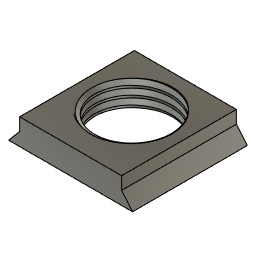
Headset_Hanger_V1.5_Fusion_v2 (Autodesk Fusion 360 archive; units mm, degrees)
design "Headset Hanger Thread"
Autodesk Fusion 360 part; units mm, degrees
sketch "Sketch1" plane through (0, 0, 0) normal (0, 0, 1) x (1, 0, 0)
  line L0 (0, 0) -> (40, 0)
  line L1 (40, 0) -> (40, 10)
  line L2 (40, 10) -> (0, 10)
  line L3 (0, 10) -> (0, 55)
  line L4 (0, 55) -> (40, 55)
  line L5 (40, 55) -> (40, 65)
  line L6 (40, 65) -> (-10, 65)
  line L7 (-10, 65) -> (-10, 0)
  line L8 (-10, 0) -> (0, 0)
  dimension "d1" = 40
  dimension "d2" = 10
  dimension "d3" = 40
  dimension "d4" = 45
  dimension "d5" = 40
  dimension "d6" = 10
  dimension "d7" = 50
  constraint coincident L0.start L8.end
  constraint horizontal L0
  constraint perpendicular L0 L1
  constraint perpendicular L1 L2
  constraint perpendicular L2 L3
  constraint perpendicular L3 L4
  constraint perpendicular L4 L5
  constraint perpendicular L3 L6
  constraint perpendicular L0 L7
  constraint perpendicular L7 L8
  measures "d1" distance of L0.start L0.end
  measures "d2" distance of L0.end L1.end
  measures "d3" distance of L1.end L2.end
  measures "d4" distance of L2.end L3.end
  measures "d5" distance of L3.end L4.end
  measures "d6" distance of L4.end L5.end
  measures "d7" distance of L5.end L6.end
sketch "Sketch2" plane through (0, 0, 30) normal (0, 0, 1) x (-1, 0, 0)
  line L0 (10, 0) -> (-40, 0)
  line L1 (-40, 0) -> (-40, -10)
  line L2 (-40, -10) -> (0, -10)
  line L3 (0, -10) -> (0, -55)
  line L4 (0, -55) -> (-40, -55)
  line L5 (-40, -55) -> (-40, -65)
  line L6 (-40, -65) -> (10, -65)
sketch "Sketch3" plane through (0, 0, 0) normal (0, 0, -1) x (1, 0, 0)
  line L0 (40, 0) -> (-10, 0)
  line L1 (-10, 0) -> (-10, -65)
  line L2 (-10, -65) -> (40, -65)
  line L3 (40, -65) -> (40, -55)
  line L4 (40, -55) -> (0, -55)
  line L5 (0, -55) -> (0, -10)
  line L6 (0, -10) -> (40, -10)
  line L7 (40, -10) -> (40, 0)
  line L8 (40, 0) -> (32, 0)
  line L9 (32, 0) -> (32, -3)
  line L10 (32, -3) -> (34.5712, -6.0642)
  line L11 (0, 0) -> (8, 0)
  line L12 (8, 0) -> (8, -3)
  line L13 (8, -3) -> (5.4288, -6.0642)
  line L14 (8, -3) -> (4, -3) construction
  line L15 (5.4288, -6.0642) -> (34.5712, -6.0642)
  dimension "d10" = 8
  dimension "d11" = 3
  dimension "d12" = 40
  dimension "d13" = 4
  dimension "d14" = 8
  dimension "d15" = 3
  dimension "d16" = 50
  dimension "d17" = 4
  constraint coincident L0.start L7.end
  constraint perpendicular L7 L8
  constraint perpendicular L0 L9
  constraint coincident L11.start origin
  constraint parallel L0 L11
  constraint perpendicular L0 L12
  constraint horizontal L14
  measures "d10" distance of L0.start L8.end
  measures "d11" distance of L8.end L9.end
  measures "d12" angle of L9 L10
  measures "d13" distance of L9.end L10.end
  measures "d14" distance of L11.start L11.end
  measures "d15" distance of L11.end L12.end
  measures "d16" angle of L13 L14
  measures "d17" distance of L12.end L13.end
sketch "Sketch4" plane through (0, 10, 0) normal (0, 1, 0) x (-1, 0, 0)
  line L0 (-40, 0) -> (0, 0)
  line L1 (0, 0) -> (0, 30)
  line L2 (0, 30) -> (-40, 30)
  line L3 (-40, 30) -> (-40, 0)
  line L4 (-20, 30) -> (-20, 15)
  circle A0 centre (-20, 15) radius 11
  dimension "d20" = 15
  dimension "d21" = 22
  constraint midpoint L2 L4.start
  constraint perpendicular L0 L4
  constraint coincident L4.end A0.centre
  measures "d20" distance of L4.start L4.end
  measures "d21" diameter of A0
sketch "Sketch5" plane through (0, 0, 0) normal (0, 0, 1) x (1, 0, 0)
  line L0 (-34.0777, 0) -> (-34.0777, 3)
  line L1 (-34.0777, 3) -> (-31.5066, 6.0642)
  line L2 (-34.0777, 3) -> (-30.0777, 3) construction
  line L3 (-58.0777, 0) -> (-58.0777, 3)
  line L4 (-58.0777, 3) -> (-60.6489, 6.0642)
  line L5 (-60.6489, 6.0642) -> (-31.5066, 6.0642)
  line L6 (-34.0777, 0) -> (-58.0777, 0)
  dimension "d26" = 3
  dimension "d27" = 4
  dimension "d28" = 50
  dimension "d30" = 3
  dimension "d31" = 140
  dimension "d32" = 4
  constraint horizontal L2
  constraint perpendicular L3 L6
  measures "d26" distance of L0.start L0.end
  measures "d27" distance of L0.end L1.end
  measures "d28" angle of L1 L2
  measures "d30" distance of L3.start L3.end
  measures "d31" angle of L3 L4
  measures "d32" distance of L3.end L4.end
extrude "Extrude4" add sketch "Sketch5" along normal blind 30
sketch "Sketch6" plane through (0, 0, 0) normal (0, -1, 0) x (1, 0, 0)
  line L0 (-58.0777, 0) -> (-34.0777, 0)
  line L1 (-34.0777, 0) -> (-34.0777, 30)
  line L2 (-34.0777, 30) -> (-58.0777, 30)
  line L3 (-58.0777, 30) -> (-58.0777, 0)
  line L4 (-58.0777, 30) -> (-34.0777, 0)
  circle A0 centre (-46.0777, 15) radius 10
  dimension "d35" = 20
  constraint coincident L2.end L3.start
  constraint coincident L0.end L1.start
  constraint midpoint L4 A0.centre
  measures "d35" diameter of A0
extrude "Extrude5" cut sketch "Sketch6" against normal blind 15 contours L4 A0 | L4 A0
extrude "Extrude6" cut 1 faces at (-50.0777, 5.0428, 30) along direction (0, 0, -1) blind 3
sketch "Sketch7" plane through (-10, 0, 0) normal (-1, 0, 0) x (0, -1, 0)
  line L0 (-60, 30) -> (-60, 0)
  line L1 (-60, 0) -> (-5, 0)
  line L2 (-5, 0) -> (-5, 30)
  line L3 (-5, 30) -> (-60, 30)
  line L4 (-32.5, 30) -> (-37.5, 30)
  line L5 (-37.5, 30) -> (-37.5, 0)
  line L6 (-32.5, 30) -> (-27.5, 30)
  line L7 (-27.5, 30) -> (-27.5, 0)
  dimension "d48" = 5
  dimension "d49" = 5
  constraint midpoint L3 L4.start
  constraint parallel L3 L4
  constraint coincident L1 L5.end
  constraint perpendicular L1 L5
  constraint coincident L3 L6.end
  constraint perpendicular L3 L7
  measures "d48" distance of L4.start L4.end
  measures "d49" distance of L4.start L6.end
move_body "Move1" bodies 1 to x (1, 0, 0) y (0, 1, 0) z (0, 0, 1) at (-90, 0, 0)
sketch "Sketch8" plane through (0, 10, 0) normal (0, 1, 0) x (-1, 0, 0)
  line L0 (10, 0) -> (65, 0)
  line L1 (65, 0) -> (65, 30)
  line L2 (65, 30) -> (10, 30)
  line L3 (65, 0) -> (55, 0)
  line L4 (55, 0) -> (55, 30)
  line L5 (10, 30) -> (10, 0)
  dimension "d62" = 10
  constraint coincident L0.end L1.start
  constraint perpendicular L1 L3
  constraint coincident L2 L4.end
  constraint perpendicular L2 L4
  measures "d62" distance of L0.end L3.end
move_body "Move2" bodies 1 to x (1, 0, 0) y (0, 0, -1) z (0, 1, 0) at (0, -19.8449, 19.8449)
move_body "Move3" bodies 1 to x (1, 0, 0) y (0, 1, 0) z (0, 0, 1) at (100, 40, 0)
move_body "Align1" bodies 1 to x (1, 0, 0) y (0, 1, 0) z (0, 0, 1) at (26.0777, -35.1551, 16.2193)
move_body "Align2" bodies 1 to x (1, 0, 0) y (0, 1, 0) z (0, 0, 1) at (0, 0, -30)
move_body "Move4" bodies 1 to x (1, 0, 0) y (0, 1, 0) z (0, 0, 1) at (-31, 40, 0)
move_body "Move5" bodies 1 to x (1, 0, 0) y (0, 1, 0) z (0, 0, 1) at (7, -4, 0)
thread "Thread2" "ISO Metric profile 20.0 M20x2 6H" major diameter 20.2503 minor diameter 18.0224 pitch 2 angle 60 modelled right hand crest width 0.547 on face at (-24.0497, 36.9957, 2.0214) crest through (-24.9888, 36, 5.5642)
named bodies: "Thread"
